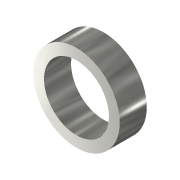
# Autodesk Inventor part: 00_Ballbearing_3x8mm
Saved by Autodesk Inventor 2022 (Build 260153000, 153)
## iProperties
Created: 2022-02-14
Part Number: 00_Ballbearing_3x8mm
Material: Generisch
Document SubType Name: Modeling
Designer: diederichbenedict
Density: 1 g/cm^3
Appearance: Silber
Author: diederichbenedict
Autodesk Inventor part; units mm, degrees
ref_plane "YZ Plane" through (0, 0, 0) normal (1, 0, 0) x (0, 1, 0)
ref_plane "XZ Plane" through (0, 0, 0) normal (0, 1, 0) x (-1, 0, 0)
ref_plane "XY Plane" through (0, 0, 0) normal (0, 0, 1) x (1, 0, 0)
sketch "Skizze1" plane through (0, 0, 0) normal (0, 0, 1) x (1, 0, 0)
  circle A0 centre (0, 0) radius 2.5 projected
  circle A1 centre (0, 0) radius 3 projected
  circle A2 centre (0, 0) radius 2.5
  circle A3 centre (0, 0) radius 4
  point P0 (0, 0)
  dimension "d0" = 8
  constraints: 2 centre point, 2 coincident, 1 concentric
  measures "d0" diameter of A3
extrude "Extrusion1" add sketch "Skizze1" along normal blind 2.5 contours A1 | A3
